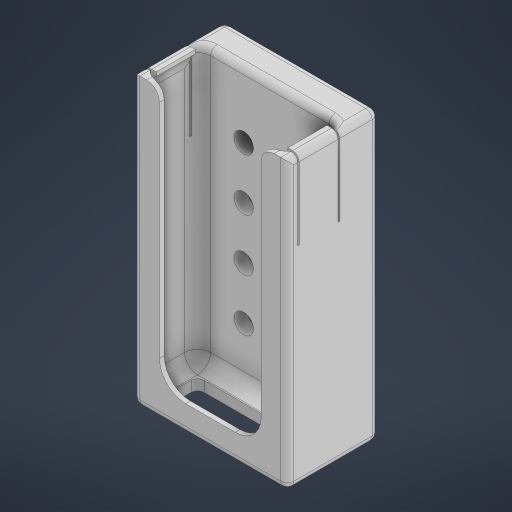
# Autodesk Inventor part: iniu_battery_mount-003
Saved by Autodesk Inventor 2023 (Build 270158000, 158)
## iProperties
Created: 2024-02-26
Part Number: iniu_battery_mount-003
Material: Generic
Document SubType Name: Modeling
Designer: Paul
Density: 1 g/cm^3
Appearance: Default
Author: Paul
Autodesk Inventor part; units mm, degrees
ref_plane "YZ Plane" through (0, 0, 0) normal (1, 0, 0) x (0, 1, 0)
ref_plane "XZ Plane" through (0, 0, 0) normal (0, 1, 0) x (-1, 0, 0)
ref_plane "XY Plane" through (0, 0, 0) normal (0, 0, 1) x (1, 0, 0)
sketch "Sketch1" plane through (0, 0, 0) normal (0, 0, 1) x (1, 0, 0)
  line L0 (-34.925, -67.31) -> (34.925, -67.31) construction
  line L1 (34.925, -67.31) -> (34.925, 67.31) construction
  line L2 (34.925, 67.31) -> (-34.925, 67.31) construction
  line L3 (-34.925, 67.31) -> (-34.925, -67.31) construction
  line L4 (-34.925, -67.31) -> (34.925, 67.31) construction
  line L5 (34.925, -67.31) -> (-34.925, 67.31) construction
  line L6 (37.465, -69.85) -> (-37.465, -69.85)
  line L7 (-37.465, -69.85) -> (-37.465, 69.85)
  line L8 (-37.465, 69.85) -> (37.465, 69.85)
  line L9 (37.465, 69.85) -> (37.465, -69.85)
  point P0 (0, 0)
  dimension "d0" = 69.85
  dimension "d1" = 134.62
  dimension "d2" = 2.54
  constraints: 20 end point, 4 parallel, 2 midpoint, 2 perpendicular, 1 horizontal, 3 other
  measures "d0" distance of L1.end L2.end
  measures "d1" distance of L0.end L1.end
  measures "d2" distance between parallel lines of L0 L6
extrude "Extrusion1" add sketch "Sketch1" along normal blind 44.45
sketch "Sketch2" plane through (-37.465, 69.85, 0) normal (0, 1, 0) x (1, 0, 0)
  line L0 (2.286, -42.164) -> (72.644, -42.164)
  line L1 (72.644, -42.164) -> (72.644, -15.494)
  line L2 (72.644, -15.494) -> (2.286, -15.494)
  line L3 (2.286, -15.494) -> (2.286, -42.164)
  line L4 (74.93, -44.45) -> (0, -44.45) projected
  line L5 (0, 0) -> (0, -44.45) projected
  line L6 (74.93, 0) -> (74.93, -44.45) projected
  point P0 (37.465, 0)
  dimension "d5" = 2.286
  dimension "d6" = 2.286
  dimension "d7" = 2.286
  dimension "d8" = 26.67
  constraints: 8 end point, 2 parallel, 1 horizontal, 1 perpendicular
  measures "d5" distance between parallel lines of L4 L0
  measures "d6" distance between parallel lines of L5 L3
  measures "d7" distance between parallel lines of L6 L1
  measures "d8" distance between parallel lines of L0 L2
extrude "Extrusion2" cut sketch "Sketch2" against normal blind 134.62
sketch "Sketch3" plane through (0, 0, 44.45) normal (0, 0, 1) x (1, 0, 0)
  line L0 (37.465, 69.85) -> (-37.465, 69.85) projected
  line L1 (-24.765, 69.85) -> (24.765, 69.85)
  line L2 (24.765, 69.85) -> (24.765, -57.15)
  line L3 (24.765, -57.15) -> (-24.765, -57.15)
  line L4 (-24.765, -57.15) -> (-24.765, 69.85)
  line L5 (-37.465, 69.85) -> (-37.465, -69.85) projected
  line L6 (37.465, -69.85) -> (37.465, 69.85) projected
  line L7 (-37.465, -69.85) -> (37.465, -69.85) projected
  point P0 (0, 0)
  dimension "d11" = 12.7
  dimension "d12" = 12.7
  dimension "d13" = 12.7
  constraints: 8 end point, 2 parallel, 1 horizontal, 1 perpendicular, 1 point on line
  measures "d11" distance between parallel lines of L5 L4
  measures "d12" distance between parallel lines of L6 L2
  measures "d13" distance between parallel lines of L7 L3
extrude "Extrusion3" cut sketch "Sketch3" against normal up to surface (2.286 mm away) contours L2 L3 L4 L0
fillet "Fillet1" radius 6.35 8 edges at (-35.179, 2.54, 15.494) (-35.179, 2.54, 42.164) (35.179, 2.54, 42.164) (35.179, 2.54, 15.494) (35.179, -64.77, 28.829) (-35.179, -64.77, 28.829) (0, -64.77, 15.494) (0, -64.77, 42.164)
sketch "Sketch4" plane through (37.465, -69.85, 0) normal (1, 0, 0) x (0, 0, -1)
  line L0 (0, 139.7) -> (-44.45, 139.7) projected
  line L1 (-39.37, 139.7) -> (-38.735, 139.7)
  line L2 (-38.735, 139.7) -> (-38.735, 101.6)
  line L3 (-38.735, 101.6) -> (-39.37, 101.6)
  line L4 (-39.37, 101.6) -> (-39.37, 139.7)
  line L5 (-19.685, 139.7) -> (-19.05, 139.7)
  line L6 (-19.05, 139.7) -> (-19.05, 101.6)
  line L7 (-19.05, 101.6) -> (-19.685, 101.6)
  line L8 (-19.685, 101.6) -> (-19.685, 139.7)
  line L9 (-44.45, 0) -> (-44.45, 139.7) projected
  point P0 (0, 69.85)
  dimension "d17" = 5.08
  dimension "d18" = 0.635
  dimension "d19" = 0.635
  dimension "d20" = 19.05
  dimension "d21" = 38.1
  constraints: 16 end point, 4 parallel, 3 point on line, 2 horizontal, 2 perpendicular
  measures "d17" distance between parallel lines of L9 L4
  measures "d18" distance between parallel lines of L4 L2
  measures "d19" distance between parallel lines of L8 L6
  measures "d20" distance between parallel lines of L8 L2
  measures "d21" distance of L3.end L1.start
extrude "Extrusion4" cut sketch "Sketch4" against normal through all
sketch "Sketch5" plane through (-37.465, 69.85, 38.735) normal (0, 0, 1) x (1, 0, 0)
  line L0 (0, 0) -> (0, -139.7) projected
  line L1 (2.9337, 0) -> (2.9337, -38.1) construction
  line L2 (2.286, -128.27) -> (2.286, 0) projected
  line L3 (2.286, 0) -> (2.286, -128.27) projected
  line L4 (5.461, -127) -> (5.461, 0)
  arc A0 (5.461, -1.905) -> (2.286, -9.525) centre (11.7974, -9.0166) ccw
  line L5 (2.6643, 0) -> (0, 0) projected
  line L6 (2.286, 0) -> (5.461, 0)
  line L7 (8.636, 0) -> (2.9337, 0) construction
  point P0 (37.465, -69.85)
  point P1 (5.461, -0.635)
  point P2 (2.286, -9.525)
  point P3 (2.286, 0)
  point P4 (2.286, -8.5083)
  dimension "d32" = 3.175
  dimension "d33" = 1.27
  dimension "d35" = 9.525
  dimension "d36" = 9.525
  dimension "d37" = 0.635
  constraints: 4 end point, 3 point on line, 2 point on circle, 1 centre point, 1 collinear, 1 parallel
  measures "d32" distance between parallel lines of L2 L4
  measures "d33" distance of A0.start point (5.461, -0.635)
  measures "d35" radius of A0
  measures "d36" distance from line of L5 A0.end
  measures "d37" distance of L4.end point (5.461, -0.635)
extrude "Extrusion5" add sketch "Sketch5" against normal up to surface (19.05 mm away) contours L2 L5 L6 L4 A0
mirror "Mirror1" about plane through (0, 0, 0) normal (1, 0, 0) of "Extrusion5"
sketch "Sketch6" plane through (-37.465, -69.85, 0) normal (0, -1, 0) x (1, 0, 0)
  line L0 (66.294, 35.814) -> (8.636, 35.814) construction
  line L1 (66.294, 21.844) -> (66.294, 35.814) construction
  line L2 (8.636, 21.844) -> (66.294, 21.844) construction
  line L3 (8.636, 35.814) -> (8.636, 21.844) construction
  line L4 (9.271, 35.179) -> (65.659, 35.179)
  line L5 (65.659, 35.179) -> (65.659, 22.479)
  line L6 (65.659, 22.479) -> (9.271, 22.479)
  line L7 (9.271, 22.479) -> (9.271, 35.179)
  point P0 (37.465, 0)
  dimension "d38" = 0.635
  constraints: 8 end point, 3 other
  measures "d38" distance between parallel lines of L0 L4
extrude "Extrusion6" cut sketch "Sketch6" against normal blind 25.4
sketch "Sketch7" plane through (-28.829, 69.85, 15.494) normal (0, 0, 1) x (1, 0, 0)
  line L0 (-8.636, 0) -> (-8.636, -139.7) projected
  line L1 (0, 0) -> (57.658, 0) construction
  line L2 (28.829, 0) -> (28.829, -139.7) construction
  line L3 (-8.636, -139.7) -> (66.294, -139.7) construction
  line L4 (-8.636, -69.85) -> (66.294, -69.85) construction
  point P0 (28.829, -69.85)
  point P1 (16.129, -31.75)
  dimension "d42" = 12.7
  dimension "d43" = 38.1
  constraints: 4 end point, 3 midpoint, 1 horizontal
  measures "d42" distance from line of L2 point (16.129, -31.75)
  measures "d43" distance from line of point (16.129, -31.75) L4
hole "Hole1" at (-12.7, 38.1, 15.494) direction (0, 0, -1) diameter 3.9624 end through all counterbore diameter 9.525 counterbore depth 6.35 thread size "10-32 UNF" class "2B" standard "ANSI Unified Screw Threads"
pattern_linear "Rectangular Pattern1" count 2 spacing 25.4 along (1, 0, 0) count 4 spacing 25.4 along (0, -1, 0) of "Hole1"
fillet "Fillet2" radius 12.7 2 edges at (-24.765, -57.15, 43.307) (24.765, -57.15, 43.307)
fillet "Fillet3" radius 6.35 2 edges at (-24.765, 69.85, 43.307) (24.765, 69.85, 43.307)
fillet "Fillet4" radius 3.175 22 edges at (37.465, 0, 44.45) (37.465, 0, 0) (-37.465, 0, 44.45) (-37.465, 0, 0) (0, 69.85, 0) (37.465, 69.85, 41.91) (37.465, 69.85, 29.21) (37.465, 69.85, 9.525) (-37.465, 69.85, 41.91) (-37.465, 69.85, 29.21) (-37.465, 69.85, 9.525) (0, 69.85, 15.494) (-32.1891, 69.85, 16.4558) (32.1891, 69.85, 16.4558) (0, -69.85, 44.45) (-37.465, -69.85, 22.225) (0, -69.85, 0) (37.465, -69.85, 22.225) (-28.194, -67.31, 35.179) (-28.194, -67.31, 22.479) (28.194, -67.31, 22.479) (28.194, -67.31, 35.179)
equation "\"d6\" = d5"
equation "\"d7\" = d5"
equation "\"d12\" = d11"
equation "\"d13\" = d11"
equation "\"d19\" = d18"
body "Solid1"
